Autodesk Fusion 360 part; units mm, degrees
(part 2 of 2)
  constraint coincident L48 L149.end
  constraint parallel L148 L149
  constraint coincident L65 L150.start
  constraint coincident L73 L150.end
  constraint parallel L149 L150
  constraint coincident L65 L151.start
  constraint coincident L73 L151.end
  constraint coincident L65 L152.start
  constraint coincident L73 L152.end
  constraint parallel L151 L152
  constraint parallel L150 L152
  constraint midpoint L147 L153.start
  constraint midpoint L148 L153.end
  constraint midpoint L149 L154.end
  constraint midpoint L150 L155.end
  constraint midpoint L152 L156.end
  constraint midpoint L151 L157.end
  constraint equal L153 L154
  constraint equal L154 L155
  constraint equal L155 L156
  constraint equal L156 L157
  constraint equal L158 L159
  constraint equal L157 L158
  constraint coincident L61 L250.start
  constraint coincident L74 L250.end
  constraint coincident L74 L251.start
  constraint coincident L61 L251.end
  constraint parallel L250 L251
  constraint coincident L74 L252.start
  constraint coincident L61 L252.end
  constraint coincident L91 L253.start
  constraint coincident L67 L253.end
  constraint parallel L252 L253
  constraint coincident L67 L254.start
  constraint coincident L91 L254.end
  constraint parallel L253 L254
  constraint coincident L67 L255.start
  constraint coincident L91 L255.end
  constraint parallel L254 L255
  constraint parallel L251 L252
  constraint midpoint L250 L256.start
  constraint midpoint L251 L256.end
  constraint midpoint L252 L257.end
  constraint midpoint L255 L258.end
  constraint midpoint L254 L259.end
  constraint midpoint L253 L260.end
  constraint equal L256 L262
  constraint equal L256 L257
  constraint equal L260 L261
  constraint equal L259 L260
  constraint equal L258 L259
  constraint equal L257 L258
  constraint midpoint L113 L353.start
  constraint perpendicular L113 L353
  constraint midpoint L16 L354.end
  constraint perpendicular L16 L354
  constraint coincident L353.end L354.start
  measures "d158" distance of L16.start L16.end
  measures "d159" angle of L71 L147
  measures "d164" angle of L74 L250
  measures "d169" diameter of A4
sketch "Sketch1 (9)" plane through (0, 0, 8.6) normal (0, 0, 1) x (-1, 0, 0) in component "SwitchShim"
  circle A0 centre (-131, 153.5) radius 1.6
  circle A1 centre (131, -153.5) radius 2.6
  circle A2 centre (-131, -153.5) radius 1.6
  circle A3 centre (131, 153.5) radius 1.6
  line L0 (48, 101.858) -> (-48, 101.858)
  line L1 (-48, 101.858) -> (-48, 153.858)
  line L2 (-48, 153.858) -> (48, 153.858)
  line L3 (48, 153.858) -> (48, 101.858)
  line L4 (67.975, 134.883) -> (82.025, 134.883)
  line L5 (82.025, 134.883) -> (82.025, 120.833)
  line L6 (82.025, 120.833) -> (67.975, 120.833)
  line L7 (67.975, 120.833) -> (67.975, 134.883)
  line L8 (135.6, -158.1) -> (135.6, 158.1)
  line L9 (135.6, 158.1) -> (-135.6, 158.1)
  line L10 (-135.6, 158.1) -> (-135.6, -158.1)
  line L11 (-135.6, -158.1) -> (135.6, -158.1)
  line L12 (59.975, 142.883) -> (90.025, 142.883)
  line L13 (90.025, 142.883) -> (90.025, 112.833)
  line L14 (90.025, 112.833) -> (59.975, 112.833)
  line L15 (59.975, 112.833) -> (59.975, 142.883)
  line L16 (67.475, 135.383) -> (82.525, 135.383)
  line L17 (82.525, 135.383) -> (82.525, 120.333)
  line L18 (82.525, 120.333) -> (67.475, 120.333)
  line L19 (67.475, 120.333) -> (67.475, 135.383)
  dimension "d175" = -8
  dimension "d176" = -0.5
extrude "Extrude1''''''''" add sketch "Sketch1 (9)" along normal blind 4 separate body contours L12 L13 L14 L15 makes body 9 in component "SwitchShim"
sketch "Sketch1 (10)" plane through (0, 0, 8.6) normal (0, 0, 1) x (-1, 0, 0) in component "ScreenCover"
  circle A0 centre (-131, 153.5) radius 1.6
  line L0 (48, 101.858) -> (-48, 101.858)
  line L1 (-48, 101.858) -> (-48, 153.858)
  line L2 (-48, 153.858) -> (48, 153.858)
  line L3 (48, 153.858) -> (48, 101.858)
  circle A1 centre (131, 153.5) radius 1.6
  circle A2 centre (-131, -153.5) radius 1.6
  circle A3 centre (131, -153.5) radius 2.6
  line L4 (67.975, 134.883) -> (82.025, 134.883)
  line L5 (82.025, 134.883) -> (82.025, 120.833)
  line L6 (82.025, 120.833) -> (67.975, 120.833)
  line L7 (67.975, 120.833) -> (67.975, 134.883)
  line L8 (135.6, -158.1) -> (135.6, 158.1)
  line L9 (135.6, 158.1) -> (-135.6, 158.1)
  line L10 (-135.6, 158.1) -> (-135.6, -158.1)
  line L11 (-135.6, -158.1) -> (135.6, -158.1)
  line L12 (47.75, 153.608) -> (47.75, 102.108)
  line L13 (47.75, 102.108) -> (-47.75, 102.108)
  line L14 (-47.75, 102.108) -> (-47.75, 153.608)
  line L15 (-47.75, 153.608) -> (47.75, 153.608)
  line L16 (-47.75, 153.608) -> (-47.75, 158.1)
  line L17 (47.75, 153.608) -> (47.75, 158.1)
  line L18 (43, 102.108) -> (43, 153.608)
  line L19 (-43, 102.108) -> (-43, 153.608)
  line L20 (-43, 127.858) -> (-47.75, 127.858) construction
  line L21 (43, 127.858) -> (47.75, 127.858) construction
  line L22 (43, 106.858) -> (-43, 106.858)
  line L23 (0, 102.108) -> (0, 106.858) construction
  line L24 (43, 148.858) -> (-43, 148.858)
  line L25 (0, 148.858) -> (0, 153.608) construction
  dimension "d199" = 0.25
  dimension "d200" = 5
  constraint coincident L9 L16.end
  constraint perpendicular L9 L16
  constraint perpendicular L15 L17
  constraint coincident L9 L17.end
  constraint coincident L13 L18.start
  constraint coincident L15 L18.end
  constraint perpendicular L15 L18
  constraint coincident L13 L19.start
  constraint coincident L15 L19.end
  constraint perpendicular L15 L19
  constraint midpoint L19 L20.start
  constraint midpoint L14 L20.end
  constraint midpoint L18 L21.start
  constraint midpoint L12 L21.end
  constraint equal L20 L21
  constraint coincident L18 L22.start
  constraint coincident L19 L22.end
  constraint perpendicular L19 L22
  constraint midpoint L13 L23.start
  constraint midpoint L22 L23.end
  constraint equal L20 L23
  constraint coincident L18 L24.start
  constraint coincident L19 L24.end
  constraint perpendicular L19 L24
  constraint midpoint L24 L25.start
  constraint midpoint L15 L25.end
  constraint equal L23 L25
  measures "d200" distance of L1 L19
extrude "Extrude1'''''''''" add sketch "Sketch1 (10)" along normal blind 4 separate body contours L2 L15 L16 L17 | L2 L9 L16 L17 | L12 L13 L15 L18 | L13 L14 L15 L19 | L15 L18 L19 L24 | L13 L18 L19 L22 makes body 10 in component "ScreenCover"
ref_plane "WorkPlane1" through (0, -130.104, 17.02) normal (0, 0, 1) x (1, 0, 0) in component "ScreenCover"
sketch "Sketch2 (3)" plane through (0, -130.104, 17.02) normal (0, 0, 1) x (1, 0, 0) in component "ScreenCover"
  line L0 (-36.5, -10.354) -> (-36.5, 14.846)
  line L1 (-36.5, 14.846) -> (36.5, 14.846)
  line L2 (36.5, -10.354) -> (-36.5, -10.354)
  line L3 (36.5, 14.846) -> (36.5, -10.354)
  line L4 (40, 20.246) -> (40, -15.754)
  line L5 (-40, 20.246) -> (40, 20.246)
  line L6 (-40, -15.754) -> (-40, 20.246)
  line L7 (40, -15.754) -> (-40, -15.754)
  line L8 (-43, -18.754) -> (-43, 23.246)
  line L9 (-43, 23.246) -> (43, 23.246)
  line L10 (43, 23.246) -> (43, -18.754)
  line L11 (43, -18.754) -> (-43, -18.754)
  line L12 (-47.75, 27.996) -> (-47.75, -27.996)
  line L13 (-47.75, -27.996) -> (47.75, -27.996)
  line L14 (47.75, -27.996) -> (47.75, 27.996)
  line L15 (47.75, 27.996) -> (-47.75, 27.996)
  line L16 (47.75, -23.504) -> (-47.75, -23.504)
extrude "Extrude2''" add sketch "Sketch2 (3)" along normal blind 3 separate body contours L8 L9 L10 L11 | L12 L14 L15 L16 makes body 11 in component "ScreenCover"
extrude "Extrude3''" add sketch "Sketch2 (3)" against normal up to surface (4.42 mm away) contours L12 L14 L15 L16 bodies 10 11 in component "ScreenCover"
sketch "Sketch3 (3)" plane through (0, 0, 8.6) normal (0, 0, -1) x (1, 0, 0) in component "ScreenCover"
  line L0 (-43, 106.858) -> (-43, 148.858)
  line L1 (-43, 148.858) -> (43, 148.858)
  line L2 (43, 148.858) -> (43, 106.858)
  line L3 (43, 106.858) -> (-43, 106.858)
  line L4 (-47.75, 158.1) -> (-47.75, 102.108)
  line L5 (-47.75, 102.108) -> (47.75, 102.108)
  line L6 (47.75, 102.108) -> (47.75, 158.1)
  line L7 (47.75, 158.1) -> (-47.75, 158.1)
  line L8 (0, 102.108) -> (0, 92.108) construction
  line L9 (0, 92.108) -> (8, 92.108)
  line L10 (8, 92.108) -> (8, 102.108)
  line L11 (0, 92.108) -> (-8, 92.108)
  line L12 (-8, 92.108) -> (-8, 102.108)
  line L13 (0, 102.108) -> (0, 106.858) construction
  line L14 (0, 104.483) -> (-15, 104.483) construction
  line L15 (-15, 102.108) -> (-15, 106.858) construction
  line L16 (-11, 106.858) -> (-11, 102.108)
  line L17 (-19, 106.858) -> (-19, 102.108)
  line L18 (-15, 104.483) -> (-45, 104.483) construction
  line L19 (-43, 106.858) -> (-47.75, 106.858)
  line L20 (-45, 102.108) -> (-45, 106.858) construction
  line L21 (-41, 106.858) -> (-41, 102.108)
  line L22 (-11, 104.108) -> (-19, 104.108)
  line L23 (-41, 104.108) -> (-47.75, 104.108)
  line L24 (11, 106.858) -> (11, 102.108)
  line L25 (11, 104.108) -> (19, 104.108)
  line L26 (19, 106.858) -> (19, 102.108)
  line L27 (41, 106.858) -> (41, 102.108)
  line L28 (41, 104.108) -> (47.75, 104.108)
  line L29 (43, 106.858) -> (-43, 148.858) construction
  line L30 (-43, 106.858) -> (43, 148.858) construction
  line L31 (0, 127.858) -> (45, 127.858) construction
  line L32 (49, 121.608) -> (41, 121.608)
  line L33 (41, 121.608) -> (41, 134.108)
  line L34 (41, 134.108) -> (49, 134.108)
  line L35 (49, 134.108) -> (49, 121.608)
  line L36 (49, 121.608) -> (41, 134.108) construction
  line L37 (41, 121.608) -> (49, 134.108) construction
  line L38 (-49, 121.608) -> (-41, 121.608)
  line L39 (-49, 134.108) -> (-49, 121.608)
  line L40 (-41, 121.608) -> (-41, 134.108)
  line L41 (-41, 134.108) -> (-49, 134.108)
  line L42 (45, 127.858) -> (45, 142.858)
  line L43 (49, 138.858) -> (41, 138.858)
  line L44 (41, 138.858) -> (41, 146.858)
  line L45 (41, 146.858) -> (49, 146.858)
  line L46 (49, 146.858) -> (49, 138.858)
  line L47 (49, 138.858) -> (41, 146.858) construction
  line L48 (41, 138.858) -> (49, 146.858) construction
  point P0 (0, 127.858)
  point P1 (45, 127.858)
  point P2 (45, 142.858)
  dimension "d210" = 8
  dimension "d211" = 10
  dimension "d212" = 15
  dimension "d213" = 4
  dimension "d214" = 30
  dimension "d215" = 4
  dimension "d216" = 2
  dimension "d217" = 2
  dimension "d222" = 45
  dimension "d223" = 8
  dimension "d224" = 12.5
  dimension "d225" = 15
  dimension "d226" = 8
  dimension "d227" = 8
  constraint midpoint L5 L8.start
  constraint perpendicular L5 L8
  constraint perpendicular L8 L9
  constraint coincident L5 L10.end
  constraint perpendicular L5 L10
  constraint symmetric L9.start L8 L11.start
  constraint symmetric L8 L9.end L11.end
  constraint symmetric L8 L10.end L12.end
  constraint midpoint L3 L13.end
  constraint midpoint L13 L14.start
  constraint perpendicular L13 L14
  constraint coincident L5 L15.start
  constraint coincident L3 L15.end
  constraint perpendicular L3 L15
  constraint coincident L14.end L15
  constraint coincident L3 L16.start
  constraint coincident L5 L16.end
  constraint perpendicular L5 L16
  constraint symmetric L15 L16.start L17.start
  constraint symmetric L15 L16.end L17.end
  constraint perpendicular L15 L18
  constraint coincident L0.start L3.end
  constraint coincident L4 L19.end
  constraint perpendicular L4 L19
  constraint coincident L5 L20.start
  constraint coincident L19 L20.end
  constraint perpendicular L19 L20
  constraint coincident L18.end L20
  constraint coincident L3 L21.start
  constraint coincident L5 L21.end
  constraint perpendicular L5 L21
  constraint coincident L16 L22.start
  constraint coincident L17 L22.end
  constraint perpendicular L17 L22
  constraint coincident L21 L23.start
  constraint coincident L4 L23.end
  constraint perpendicular L4 L23
  constraint symmetric L13 L16.start L24.start
  constraint symmetric L13 L16.end L24.end
  constraint symmetric L13 L17.start L26.start
  constraint symmetric L13 L17.end L26.end
  constraint symmetric L13 L21.start L27.start
  constraint symmetric L13 L21.end L27.end
  constraint symmetric L13 L22.start L25.start
  constraint symmetric L13 L22.end L25.end
  constraint symmetric L13 L23.start L28.start
  constraint symmetric L13 L23.end L28.end
  constraint coincident L2.end L3.start
  constraint coincident L0.end L1.start
  constraint coincident L1.end L2.start
  constraint midpoint L29 P0
  constraint coincident P0 L31.start
  constraint horizontal L31
  constraint horizontal L32
  constraint perpendicular L32 L33
  constraint parallel L32 L34
  constraint parallel L33 L35
  constraint coincident L36 P1
  constraint coincident L37 P1
  constraint coincident P1 L31.end
  constraint symmetric L13 L32.start L38.start
  constraint symmetric L13 L32.end L38.end
  constraint symmetric L13 L33.end L40.end
  constraint symmetric L13 L34.end L39.start
  constraint perpendicular L31 L42
  constraint horizontal L43
  constraint perpendicular L43 L44
  constraint parallel L43 L45
  constraint parallel L44 L46
  constraint coincident L47 P2
  constraint coincident L48 P2
  constraint coincident P2 L42.end
  measures "d210" distance of L8.end L9.end
  measures "d211" distance of L9.end L10.end
  measures "d212" distance of L14.start L14.end
  measures "d213" distance of L15.start L16.end
  measures "d214" distance of L14.end L18.end
  measures "d215" distance of L20.start L21.end
  measures "d216" distance of L5 L22
  measures "d217" distance of L5 L23
  measures "d222" distance of P0 P1
  measures "d223" distance of L33.end L34.end
  measures "d224" distance of L32.end L33.end
  measures "d225" distance of P1 P2
  measures "d226" distance of L44.end L45.end
  measures "d227" distance of L43.end L44.end
extrude "Extrude4''" add sketch "Sketch3 (3)" against normal blind 4 contours L5 L9 L10 L11 L12 bodies 10 in component "ScreenCover"
extrude "Extrude5" cut sketch "Sketch3 (3)" against normal blind 3 contours L0 L4 L38 L41 | L4 L5 L21 L23 | L5 L16 L17 L22 | L2 L6 L43 L45 | L5 L24 L25 L26 | L2 L6 L32 L34 | L5 L6 L27 L28 bodies 10 in component "ScreenCover"
sketch "Sketch4" plane through (0, 0, 12.6) normal (0, 0, 1) x (-1, 0, 0) in component "ScreenCover"
  line L0 (-8, 92.108) -> (8, 92.108)
  line L1 (8, 92.108) -> (8, 102.108)
  line L2 (8, 102.108) -> (-8, 102.108)
  line L3 (-8, 102.108) -> (-8, 92.108)
  line L4 (-47.75, 153.608) -> (47.75, 153.608)
  line L5 (47.75, 153.608) -> (47.75, 158.1)
  line L6 (47.75, 158.1) -> (-47.75, 158.1)
  line L7 (-47.75, 158.1) -> (-47.75, 153.608)
extrude "Extrude6'" cut sketch "Sketch4" against normal blind 0.3 bodies 10 in component "ScreenCover"
component "PCB" placed x (1, 0, 0) y (0, 1, 0) z (0, 0, 1) at (0, 0, 0)
component "Connectors" placed x (1, 0, 0) y (0, 1, 0) z (0, 0, 1) at (0, 0, 0)
component "Hardware" placed x (1, 0, 0) y (0, 1, 0) z (0, 0, 1) at (0, 0, 0)
component "Panels" placed x (1, 0, 0) y (0, 1, 0) z (0, 0, 1) at (0, 0, 0)
component "SwitchShim" placed x (1, 0, 0) y (0, 1, 0) z (0, 0, 1) at (-0.5, -0.5, -7)
component "ScreenCover" placed x (1, 0, 0) y (0, 1, 0) z (0, 0, 1) at (0.25, -0.25, -6.7)
component "Corner" placed x (1, 0, 0) y (0, 1, 0) z (0, 0, 1) at (-131, 153.5, -10) in component "Connectors"
component "Washer" placed x (0, -1, 0) y (1, 0, 0) z (0, 0, 1) at (131, 153.5, -1) in component "Connectors"
component "PlateWasher" placed x (1, 0, 0) y (0, 1, 0) z (0, 0, 1) at (-131, -153.5, 1.6) in component "Connectors"
component "Corner" placed x (0, -1, 0) y (1, 0, 0) z (0, 0, 1) at (131, 153.5, -10) in component "Connectors"
component "Corner" placed x (-1, 0, 0) y (0, -1, 0) z (0, 0, 1) at (131, -153.5, -10) in component "Connectors"
component "Corner" placed x (0, 1, 0) y (-1, 0, 0) z (0, 0, 1) at (-131, -153.5, -10) in component "Connectors"
component "Washer" placed x (0, 1, 0) y (-1, 0, 0) z (0, 0, 1) at (-131, -153.5, -1) in component "Connectors"
component "Washer" placed x (1, 0, 0) y (0, 1, 0) z (0, 0, 1) at (-131, 153.5, -1) in component "Connectors"
component "Washer" placed x (-1, 0, 0) y (0, -1, 0) z (0, 0, 1) at (131, -153.5, -1) in component "Connectors"
component "PlateWasher" placed x (1, 0, 0) y (0, 1, 0) z (0, 0, 1) at (131, 153.5, 1.6) in component "Connectors"
component "PlateWasher" placed x (1, 0, 0) y (0, 1, 0) z (0, 0, 1) at (-131, 153.5, 1.6) in component "Connectors"
component "PlateWasher" placed x (1, 0, 0) y (0, 1, 0) z (0, 0, 1) at (131, -153.5, 1.6) in component "Connectors"
component "Panel1" placed x (1, 0, 0) y (0, 1, 0) z (0, 0, 1) at (0, 319.2, 0) in component "Panels"
component "Panel1" placed x (1, 0, 0) y (0, 1, 0) z (0, 0, 1) at (0, 0, 0) in component "Panels"
component "Panel2" placed x (1, 0, 0) y (0, 1, 0) z (0, 0, 1) at (0, 0, 0) in component "Panels"
component "Panel3" placed x (1, 0, 0) y (0, 1, 0) z (0, 0, 1) at (0, 0, 0) in component "Panels"
component "TopPanel" placed x (1, 0, 0) y (0, 1, 0) z (0, 0, 1) at (0, 0, 0) in component "Panels"
equation "BoltHoleDiameter = 3.2 mm"
equation "HeatInsertDiameter = 4.6 mm"
equation "HeatInsertLength = 6 mm"
equation "PCBToPlate = 4 mm" comment "Distance from top of PCB to the bottom of plate"
equation "MaterialThickness = 3 mm" comment "Laser cut material thickness"
equation "d36 = 13.2 mm - 8.6 mm"
equation "d38 = ScreenHeight"
equation "WasherThickness = 1 mm" comment "Must be multiple of PCBToPlate"
equation "d41 = HeatInsertDiameter"
equation "d42 = HeatInsertDiameter * 2"
equation "d43 = HeatInsertDiameter"
equation "d44 = HeatInsertDiameter"
equation "d45 = HeatInsertLength + 3 mm"
equation "d49 = HeatInsertDiameter"
equation "d50 = -HeatInsertLength"
equation "d52 = HeatInsertDiameter"
equation "d53 = -HeatInsertLength"
equation "d55 = BoltHoleDiameter"
equation "d57 = WasherThickness"
equation "d59 = BoltHoleDiameter"
equation "d61 = PCBToPlate"
equation "d120 = MaterialThickness"
equation "d121 = MaterialThickness"
equation "d123 = BoltHoleDiameter"
equation "d129 = BoltHoleDiameter"
equation "d130 = MaterialThickness"
equation "d132 = MaterialThickness"
equation "d134 = MaterialThickness"
equation "d177 = PCBToPlate"
equation "d201 = PCBToPlate"
equation "ScreenHeight = 13.2 mm" comment "Top of PCB to top of screen"
equation "d205 = ScreenHeight - PCBToPlate - 4.78 mm"
equation "d218 = -PCBToPlate"
